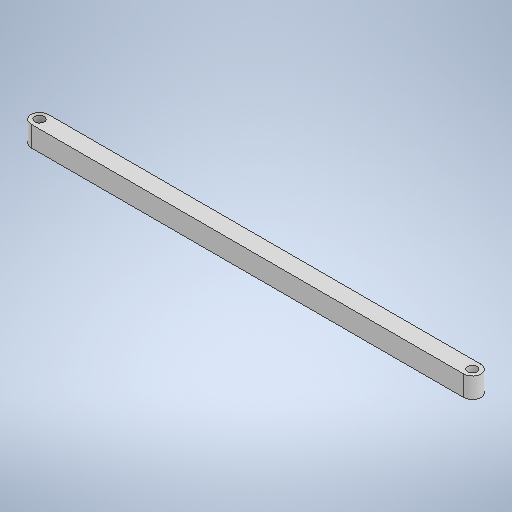
# Autodesk Inventor part: scrambler_spider_support1
Saved by Autodesk Inventor 2025.2 (Build 292293000, 293)
## iProperties
Created: 2025-10-14
Part Number: scrambler_spider_support1
Material: Generic
Document SubType Name: Modeling
Designer: pascu
Density: 1 g/cm^3
Appearance: Default
Author: pascu
Autodesk Inventor part; units mm, degrees
ref_plane "YZ Plane" through (0, 0, 0) normal (1, 0, 0) x (0, 1, 0)
ref_plane "XZ Plane" through (0, 0, 0) normal (0, 1, 0) x (-1, 0, 0)
ref_plane "XY Plane" through (0, 0, 0) normal (0, 0, 1) x (1, 0, 0)
sketch "Sketch3" plane through (0, 0, 0) normal (0, 1, 0) x (-1, 0, 0)
  circle A0 centre (0, 0) radius 0.889
  circle A1 centre (-80.7212, 0) radius 0.889
  circle A2 centre (0, 0) radius 1.5875 construction
  circle A3 centre (-80.7212, 0) radius 1.5875 construction
  line L0 (-80.7212, 1.5875) -> (0, 1.5875)
  line L1 (1.5875, 0) -> (1.5875, 0)
  line L2 (0, -1.5875) -> (-80.7212, -1.5875)
  line L3 (-82.3087, 0) -> (-82.3087, 0)
  arc A4 (0, -1.5875) -> (1.5875, 0) centre (0, 0) ccw
  arc A5 (1.5875, 0) -> (0, 1.5875) centre (0, 0) ccw
  arc A6 (-80.7212, 1.5875) -> (-82.3087, 0) centre (-80.7212, 0) ccw
  arc A7 (-82.3087, 0) -> (-80.7212, -1.5875) centre (-80.7212, 0) ccw
  dimension "d12" = 1.778
  dimension "d13" = 1.778
  dimension "d14" = 80.7212
  dimension "d15" = 3.175
  dimension "d16" = 3.175
  dimension "d17" = 1.5875
  constraints: 8 centre point, 8 end point, 8 point on circle, 8 tangent, 3 coincident, 3 equal radius, 2 parallel, 1 horizontal, 1 perpendicular
  measures "d12" diameter of A0
  measures "d13" diameter of A1
  measures "d14" distance of A1.centre point (0, 0)
  measures "d15" diameter of A2
  measures "d16" diameter of A3
  measures "d17" radius of A4
extrude "Extrusion3" add sketch "Sketch3" against normal blind 3.81
body "Solid2"
